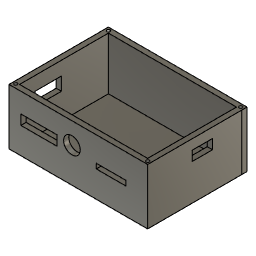
Music Player Box V1 (Autodesk Fusion 360 design; units mm, degrees)
Autodesk Fusion 360 part; units mm, degrees
note: some values were not read from the file. Set by a fixed rule: which face or edge a step refers to.
box "BoxPrimitive1" add length 2.54 width 61.9125 height 25.4 placed x (0, 1, 0) y (-1, 0, 0) z (0, 0, 1) at (61.9125, 0, 0) makes body 1
extrude "Extrude1" add 1 faces at (41.275, 0.8467, 25.4) along direction (0, 0, 1) blind 1.5875 on bodies 1 bodies 1
box "BoxPrimitive2" add length 42.8625 width 2.54 height 26.9875 placed x (0, -1, 0) y (1, 0, 0) z (0, 0, 1) at (-2.54, 0, 0) separate body makes body 2
extrude "Extrude2" add 1 faces at (-1.6933, 0, 8.9958) along direction (0, 1, 0) blind 2.54 on bodies 2 bodies 2 1
copy_body "CopyPasteBodies1" bodies 2 makes body 3
move_body "Move1" bodies 3 to x (-1, 0, 0) y (0, -1, 0) z (0, 0, 1) at (61.9104, -42.9438, 0)
extrude "Extrude3" add 1 faces at (61.9125, 0.8467, 17.9917) along direction (1, 0, 0) blind 2.5908 on bodies 2 bodies 2
extrude "Extrude4" add 1 faces at (63.6037, -0.0813, 8.9958) along direction (0, 1, 0) blind 0.1778 on bodies 3 bodies 3 2
extrude "Extrude5" cut 1 faces at (64.5033, 0.8467, 17.9917) along direction (-1, 0, 0) blind 0.0508 on bodies 3 bodies 3
extrude "Extrude6" add 1 faces at (-1.6933, -42.8625, 8.9958) along direction (0, -1, 0) blind 2.6162 on bodies 3 bodies 3
extrude "Extrude7" add 1 faces at (-0.0021, -45.4804, 17.9917) along direction (-1, 0, 0) blind 2.54 on bodies 3 bodies 3
box "BoxPrimitive3" add length 44.5594 width 64.4815 height 1.5875 placed x (0, -1, 0) y (1, 0, 0) z (0, 0, 1) at (-1.8065, 0.4087, 0) bodies 3
hole "Hole1" at (63.0686, -44.0443, 26.9875) direction (0, 0, -1) diameter 2 depth 6.477 tip angle 180 bodies 3
hole "Hole2" at (62.9235, 1.0328, 26.9875) direction (0, 0, -1) diameter 2.0066 depth 6.477 tip angle 180 bodies 3
hole "Hole3" at (-0.9818, 1.0224, 26.9875) direction (0, 0, -1) diameter 2.0066 depth 6.477 tip angle 180 bodies 3
hole "Hole4" at (-1.1057, -43.6413, 26.9875) direction (0, 0, -1) diameter 2.0066 depth 6.477 tip angle 180 bodies 3
thread "Thread1" "ANSI Unified Screw Threads 0.073(#1) 1-64 UNC 3B" major diameter 1.8542 minor diameter 1.5037 pitch 0.3969 angle 60 resizes the face on face at (-1.0557, -44.6434, 24.8285) on bodies 3
thread "Thread2" "ANSI Unified Screw Threads 0.073(#1) 1-64 UNC 3B" major diameter 1.8542 minor diameter 1.5037 pitch 0.3969 angle 60 resizes the face on face at (62.8704, -43.0641, 24.8285) on bodies 3
thread "Thread3" "ANSI Unified Screw Threads 0.073(#1) 1-64 UNC 3B" major diameter 1.8542 minor diameter 1.5037 pitch 0.3969 angle 60 resizes the face on face at (62.9735, 2.0348, 22.6695) on bodies 3
thread "Thread4" "ANSI Unified Screw Threads 0.073(#1) 1-64 UNC 3B" major diameter 1.8542 minor diameter 1.5037 pitch 0.3969 angle 60 resizes the face on face at (-0.8819, 0.024, 22.6695) on bodies 3
sketch "Sketch4" plane through (-2.54, 0, 0) normal (-1, 0, 0) x (0, -1, 0)
  line L0 (-2.54, 0) -> (45.4787, 0)
  line L1 (45.4787, 0) -> (45.4787, 26.9875)
  line L2 (45.4787, 26.9875) -> (-2.54, 26.9875)
  line L3 (-2.54, 26.9875) -> (-2.54, 0)
  line L4 (24.0518, 17.464) -> (12.9393, 17.464)
  line L5 (12.9393, 17.464) -> (12.9393, 22.1817)
  line L6 (12.9393, 22.1817) -> (24.0518, 22.1817)
  line L7 (24.0518, 22.1817) -> (24.0518, 17.464)
  dimension "d42" = 11.1125
  constraint horizontal L4
  constraint vertical L5
  constraint horizontal L6
  constraint vertical L7
  measures "d42" distance of L4.start L4.end
extrude "Extrude8" cut sketch "Sketch4" against normal blind 87.5169 contours L4 L5 L6 L7 bodies 3
sketch "Sketch5" plane through (64.4504, 0, 0) normal (1, 0, 0) x (0, 1, 0)
  line L0 (-45.4838, 0) -> (0, 0)
  line L1 (0, 0) -> (0, 26.9875)
  line L2 (0, 26.9875) -> (-45.4838, 26.9875)
  line L3 (-45.4838, 26.9875) -> (-45.4838, 0)
  line L4 (-22.7034, 20.3794) -> (-35.4034, 20.3794)
  line L5 (-35.4034, 20.3794) -> (-35.4034, 14.0019)
  line L6 (-35.4034, 14.0019) -> (-22.7034, 14.0019)
  line L7 (-22.7034, 14.0019) -> (-22.7034, 20.3794)
  line L8 (-12.9393, 22.1817) -> (-12.9393, 17.464)
  line L9 (-12.9393, 17.464) -> (-24.0518, 17.464)
  line L10 (-24.0518, 17.464) -> (-24.0518, 22.1817)
  line L11 (-24.0518, 22.1817) -> (-12.9393, 22.1817)
  dimension "d45" = 12.7
  constraint horizontal L4
  constraint vertical L5
  constraint horizontal L6
  constraint vertical L7
  measures "d45" distance of L4.start L4.end
extrude "Extrude9" cut sketch "Sketch5" against normal blind 83.8796 contours L4 L7 L9 L10 | L4 L5 L6 L7 L9 L10 bodies 3
extrude "Extrude10" add 1 faces at (-1.6933, -19.4487, 17.464) along direction (0, 0, 1) blind 6.1468 on bodies 3 bodies 3
extrude "Extrude11" add 1 faces at (-1.6933, -23.1529, 22.1817) along direction (0, 0, -1) blind 1.8034 on bodies 3 bodies 3
extrude "Extrude12" add 1 faces at (63.6037, -31.1701, 14.0019) along direction (0, 0, 1) blind 9.0932 on bodies 3 bodies 3
extrude "Extrude13" cut 1 faces at (63.6037, -22.7034, 19.0366) along direction (0, -1, 0) blind 1.1938 on bodies 3 bodies 3
extrude "Extrude14" add 1 faces at (62.7571, -12.9393, 19.0366) along direction (0, -1, 0) blind 1.1938 on bodies 3 bodies 3
sketch "Sketch6" plane through (0, -42.9438, 0) normal (0, 1, 0) x (-1, 0, 0)
  line L0 (-61.9104, 1.5875) -> (0, 1.5875)
  line L1 (0, 1.5875) -> (0, 26.9875)
  line L2 (0, 26.9875) -> (-61.9104, 26.9875)
  line L3 (-61.9104, 26.9875) -> (-61.9104, 1.5875)
  line L4 (-3.1678, 17.4807) -> (-20.6303, 17.4807)
  line L5 (-20.6303, 17.4807) -> (-20.6303, 12.6991)
  line L6 (-20.6303, 12.6991) -> (-3.1678, 12.6991)
  line L7 (-3.1678, 12.6991) -> (-3.1678, 17.4807)
  circle A0 centre (-27.8513, 16.737) radius 4.0425
  line L8 (-39.6261, 15.0764) -> (-53.9136, 15.0764)
  line L9 (-53.9136, 15.0764) -> (-53.9136, 12.6997)
  line L10 (-53.9136, 12.6997) -> (-39.6261, 12.6997)
  line L11 (-39.6261, 12.6997) -> (-39.6261, 15.0764)
  dimension "d58" = 17.4625
  dimension "d59" = 8.0851
  dimension "d60" = 14.2875
  constraint horizontal L4
  constraint vertical L5
  constraint horizontal L6
  constraint vertical L7
  constraint horizontal L8
  constraint vertical L9
  constraint horizontal L10
  constraint vertical L11
  measures "d58" distance of L4.start L4.end
  measures "d59" diameter of A0
  measures "d60" distance of L8.start L8.end
extrude "Extrude15" cut sketch "Sketch6" against normal blind 22.2504 contours L4 L5 L6 L7 | A0 | L8 L9 L10 L11 bodies 3
